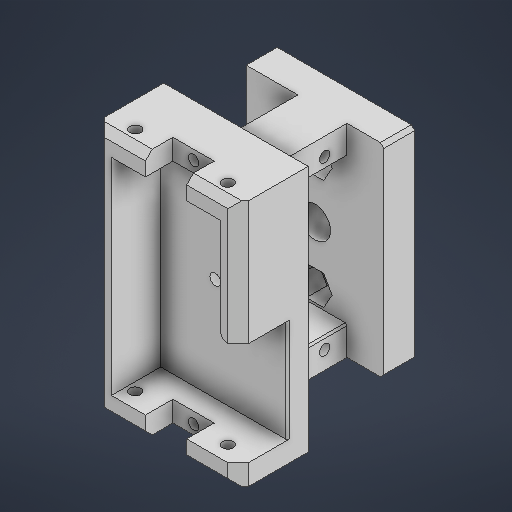
# Autodesk Inventor part: GA_Base
Saved by Autodesk Inventor 2025.2 (Build 292293000, 293)
## iProperties
Created: 2025-06-18
Part Number: GA_Base
Material: Generic
Document SubType Name: Modeling
Designer: Tiago
Density: 1 g/cm^3
Appearance: Default
Author: Tiago
Autodesk Inventor part; units mm, degrees
sketch "Sketch1" plane through (0, 0, 0) normal (0, 0, 1) x (1, 0, 0)
  line L0 (-15.9, 30) -> (15.9, 30)
  line L1 (15.9, 30) -> (15.9, -30)
  line L2 (15.9, -30) -> (-15.9, -30)
  line L3 (-15.9, -30) -> (-15.9, 30)
  line L4 (-21, -36) -> (21, -36)
  line L5 (21, -36) -> (21, 36)
  line L6 (21, 36) -> (-21, 36)
  line L7 (-21, 36) -> (-21, -36)
  circle A0 centre (0, 0) radius 1.575
  point P0 (15.9, 0)
  point P1 (0, 30)
  point P2 (0, 36)
  point P3 (-21, 0)
  dimension "d0" = 31.8
  dimension "d1" = 60
  dimension "d4" = 42
  dimension "d5" = 72
  dimension "d40" = 3.15
  constraints: 16 end point, 5 coincident, 4 midpoint, 4 parallel, 2 horizontal, 2 horizontal alignment, 2 perpendicular, 2 vertical alignment, 1 centre point
  measures "d0" distance of L1.end L2.end
  measures "d1" distance of L0.end L1.end
  measures "d4" distance of L5.end L6.end
  measures "d5" distance of L4.end L5.end
  measures "d40" diameter of A0
extrude "Extrusion1" add sketch "Sketch1" along normal blind 20.35 contours L7 L6 L5 L4
extrude "Extrusion2" add sketch "Sketch1" along normal blind 6 contours L0 L1 L2 L3
chamfer "Chamfer1" distance 3 angle 45 2 edges at (21, 0, 20.35) (-21, 0, 20.35)
chamfer "Chamfer2" distance 2 angle 45 2 edges at (0, -36, 20.35) (0, 36, 20.35)
sketch "Sketch2" plane through (0, 0, 20.35) normal (0, 0, 1) x (1, 0, 0)
  line L0 (-18, 34) -> (18, 34) projected
  line L1 (18, 34) -> (18, -34) projected
  line L2 (18, -34) -> (-18, -34) projected
  line L3 (-18, -34) -> (-18, 34) projected
  line L4 (15.9, 30) -> (-15.9, 30) projected
  line L5 (-15.9, 30) -> (-15.9, -30) projected
  line L6 (-15.9, -30) -> (15.9, -30) projected
  line L7 (15.9, -30) -> (15.9, 30) projected
  circle A0 centre (0, -33.25) radius 1.5
  line L8 (-6, -38) -> (6, -38)
  line L9 (6, -38) -> (6, -30)
  line L10 (6, -30) -> (-6, -30)
  line L11 (-6, -30) -> (-6, -38)
  line L12 (-3.2097, 0) -> (3.2097, 0) construction
  circle A1 centre (0, 33.25) radius 1.5
  line L13 (-6, 38) -> (6, 38)
  line L14 (6, 38) -> (6, 30)
  line L15 (6, 30) -> (-6, 30)
  line L16 (-6, 30) -> (-6, 38)
  point P0 (0, 0)
  point P1 (0, -30)
  point P2 (0, -30)
  point P3 (0, 0)
  point P4 (0, 30)
  point P5 (0, 30)
  dimension "d16" = 3
  dimension "d18" = 33.25
  dimension "d19" = 12
  dimension "d20" = 8
  constraints: 18 end point, 7 symmetric about line, 3 coincident, 3 midpoint, 2 centre point, 2 horizontal, 2 parallel, 2 vertical alignment, 1 perpendicular, 1 other
  measures "d16" diameter of A0
  measures "d18" distance of point (0, 0) A0.centre
  measures "d19" distance between parallel lines of L11 L9
  measures "d20" distance of L8.end L9.end
extrude "Extrusion3" cut sketch "Sketch2" against normal blind 8 contours L16 L13 L14 L0 A1 | L0 A1 L14 L4 L16 | L11 L6 L9 L2 A0 | L2 A0 L9 L8 L11
extrude "Extrusion4" cut sketch "Sketch2" against normal blind 18 contours A1 L0 | L0 A1 | A0 L2 | L2 A0
ref_plane "Work Plane1" through (15.75, -36, 0) normal (1, 0, 0) x (0, 0, -1)
sketch "Sketch4" plane through (15.75, -36, 0) normal (1, 0, 0) x (0, 0, -1)
  line L0 (-18.35, 72) -> (0, 72) projected
  line L1 (0, 72) -> (0, 0) projected
  line L2 (0, 0) -> (-18.35, 0) projected
  line L3 (-18.35, 0) -> (-20.35, 2) projected
  line L4 (-20.35, 2) -> (-20.35, 6) projected
  line L5 (-20.35, 66) -> (-20.35, 70) projected
  line L6 (-20.35, 70) -> (-18.35, 72) projected
  line L7 (-20.35, 6) -> (-6, 6)
  line L8 (-6, 6) -> (-6, 36)
  line L9 (-6, 6) -> (-6, 66) projected
  line L10 (-6, 36) -> (-20.35, 36)
  line L11 (-20.35, 36) -> (-20.35, 6)
  line L12 (-20.35, 6) -> (-6, 6) projected
  line L13 (-6, 6) -> (-6, 66) projected
  line L14 (-6, 66) -> (-20.35, 66) projected
  point P0 (0, 36)
  dimension "d26" = 30
  constraints: 8 end point, 1 collinear, 1 horizontal, 1 midpoint
  measures "d26" distance of L7.end L8.end
extrude "Extrusion5" cut sketch "Sketch4" along normal up to surface (5.25 mm away) contours L8 L7 L11 L10
fillet "Fillet1" radius 2 1 edges at (15.9, 0, 13.175)
chamfer "Chamfer3" distance 0.5 angle 45 1 edges at (21, -15, 6)
ref_plane "Work Plane2" through (-21, 33, 0) normal (0, 1, 0) x (1, 0, 0)
sketch "Sketch6" plane through (-21, 33, 0) normal (0, 1, 0) x (1, 0, 0)
  line L0 (15, -12.35) -> (15, -20.35) projected
  line L1 (15, -20.35) -> (3, -20.35) projected
  line L2 (3, -20.35) -> (0, -17.35) projected
  line L3 (0, -17.35) -> (0, 0) projected
  line L4 (0, 0) -> (42, 0) projected
  line L5 (42, 0) -> (42, -17.35) projected
  line L6 (42, -17.35) -> (39, -20.35) projected
  line L7 (39, -20.35) -> (27, -20.35) projected
  line L8 (27, -20.35) -> (27, -12.35) projected
  line L9 (27, -12.35) -> (22.479, -12.35) projected
  line L10 (22.479, -12.35) -> (22.479, -2.35) projected
  line L11 (22.479, -2.35) -> (19.521, -2.35) projected
  line L12 (19.521, -2.35) -> (19.521, -12.35) projected
  line L13 (19.521, -12.35) -> (15, -12.35) projected
  circle A0 centre (34.45, -15.85) radius 1.575
  circle A1 centre (7.55, -15.85) radius 1.575
  point P0 (21, 0)
  dimension "Veio" = 3.15
  dimension "d34" = 3.15
  dimension "d35" = 4.5
  dimension "d36" = 7.55
  dimension "d37" = 7.55
  constraints: 2 centre point, 1 horizontal alignment
  measures "Veio" diameter of A0
  measures "d34" diameter of A1
  measures "d35" distance from line of L7 A0.centre
  measures "d36" distance from line of L5 A0.centre
  measures "d37" distance from line of L3 A1.centre
extrude "Extrusion6" cut sketch "Sketch6" along normal through all both and the other way through all contours A0 | A1
sketch "Sketch7" plane through (0, 0, 0) normal (0, 0, -1) x (-1, 0, 0)
  line L0 (20, -20.5) -> (-20, -20.5)
  line L1 (-20, -20.5) -> (-20, 20.5)
  line L2 (-20, 20.5) -> (20, 20.5)
  line L3 (20, 20.5) -> (20, -20.5)
  line L4 (-9.3, -29.5) -> (20, -29.5)
  line L5 (20, -29.5) -> (20, 29.5)
  line L6 (20, 29.5) -> (-9.3, 29.5)
  line L7 (-9.3, 29.5) -> (-9.3, -29.5)
  line L8 (-9.3, -21) -> (20, -21)
  line L9 (-9.3, 21) -> (20, 21)
  line L10 (5, 29.5) -> (5, 21)
  line L11 (5, -21) -> (5, -29.5)
  point P0 (0, 0)
  point P1 (-20, 0)
  point P2 (0, -20.5)
  point P3 (20, 0)
  point P4 (20, 0)
  point P5 (-9.3, 20.5)
  point P6 (-9.3, -20.5)
  dimension "d41" = 41
  dimension "d42" = 40
  dimension "d43" = 9
  dimension "d44" = 9
  dimension "d47" = 10.7
  dimension "d101" = 0.5
  dimension "d102" = 0.5
  dimension "d122" = 15
  dimension "d123" = 15
  constraints: 24 end point, 8 point on line, 6 perpendicular, 4 midpoint, 4 parallel, 2 horizontal, 1 coincident, 1 horizontal alignment, 1 vertical alignment
  measures "d41" distance of L0.end L1.end
  measures "d42" distance of L1.end L2.end
  measures "d43" distance between parallel lines of L4 L0
  measures "d44" distance between parallel lines of L6 L2
  measures "d47" distance between parallel lines of L7 L1
  measures "d101" distance between parallel lines of L2 L9
  measures "d102" distance between parallel lines of L0 L8
  measures "d122" distance between parallel lines of L5 L11
  measures "d123" distance between parallel lines of L5 L10
extrude "Extrusion7" add sketch "Sketch7" along normal blind 23 contours L8 L11 L4 L7 | L7 L6 L10 L9
ref_plane "Work Plane3" through (0, 0, -23) normal (0, 0, -1) x (-1, 0, 0)
sketch "Sketch8" plane through (0, 0, -23) normal (0, 0, -1) x (-1, 0, 0)
  line L0 (20, -29.5) -> (-20, -29.5)
  line L1 (-20, -29.5) -> (-20, 29.5)
  line L2 (-20, 29.5) -> (20, 29.5)
  line L3 (20, 29.5) -> (20, -29.5)
  point P0 (0, 0)
  point P1 (-20, 0)
  point P2 (0, 29.5)
  dimension "d51" = 40
  dimension "d52" = 59
  constraints: 8 end point, 2 midpoint, 2 parallel, 1 horizontal, 1 horizontal alignment, 1 perpendicular, 1 vertical alignment
  measures "d51" distance of L1.end L2.end
  measures "d52" distance of L2.end L0.start
extrude "Extrusion8" add sketch "Sketch8" along normal blind 9
ref_plane "Work Plane4" through (9.3, -29.5, 0) normal (1, 0, 0) x (0, 0, -1)
sketch "Sketch9" plane through (9.3, -29.5, 0) normal (1, 0, 0) x (0, 0, -1)
  circle A0 centre (6.5, 5.2) radius 1.5
  circle A1 centre (6.5, 53.8) radius 1.5
  circle A2 centre (16.5, 53.8) radius 1.5
  circle A3 centre (16.5, 5.2) radius 1.5
  point P0 (0, 29.5)
  point P1 (11.2, 29.5)
  dimension "mss" = 3
  dimension "d57" = 3
  dimension "d58" = 3
  dimension "d59" = 3
  dimension "d60" = 24.3
  dimension "d61" = 24.3
  dimension "d62" = 24.3
  dimension "d63" = 24.3
  dimension "d64" = 10
  dimension "d65" = 10
  dimension "d66" = 11.2
  dimension "d67" = 4.7
  dimension "d68" = 4.7
  constraints: 4 centre point, 1 horizontal alignment
  measures "mss" diameter of A0
  measures "d57" diameter of A3
  measures "d58" diameter of A2
  measures "d59" diameter of A1
  measures "d60" vertical distance of A3.centre point (0, 29.5)
  measures "d61" vertical distance of point (0, 29.5) A0.centre
  measures "d62" vertical distance of point (0, 29.5) A1.centre
  measures "d63" vertical distance of point (0, 29.5) A2.centre
  measures "d64" distance of A0.centre A3.centre
  measures "d65" distance of A2.centre A1.centre
  measures "d66" distance of point (0, 29.5) point (11.2, 29.5)
  measures "d67" horizontal distance of A1.centre point (11.2, 29.5)
  measures "d68" horizontal distance of A0.centre point (11.2, 29.5)
extrude "Extrusion9" cut sketch "Sketch9" against normal through all
ref_plane "Work Plane5" through (-20, 29.5, 0) normal (0, 1, 0) x (1, 0, 0)
sketch "Sketch12" plane through (0, 0, -23) normal (0, 0, 1) x (1, 0, 0)
  circle A0 centre (0, 16) radius 2.5
  circle A1 centre (0, -16) radius 2.5
  circle A2 centre (0, 0) radius 4.5
  line L0 (-5, -16) -> (-2.5, -11.6699)
  line L1 (-2.5, -11.6699) -> (2.5, -11.6699)
  line L2 (2.5, -11.6699) -> (5, -16)
  line L3 (5, -16) -> (2.5, -20.3301)
  line L4 (2.5, -20.3301) -> (-2.5, -20.3301)
  line L5 (-2.5, -20.3301) -> (-5, -16)
  line L6 (-5, 16) -> (-2.5, 20.3301)
  line L7 (-2.5, 20.3301) -> (2.5, 20.3301)
  line L8 (2.5, 20.3301) -> (5, 16)
  line L9 (5, 16) -> (2.5, 11.6699)
  line L10 (2.5, 11.6699) -> (-2.5, 11.6699)
  line L11 (-2.5, 11.6699) -> (-5, 16)
  dimension "d103" = 32
  dimension "d104" = 5
  dimension "d105" = 5
  dimension "d106" = 9
  dimension "d107" = 16
  dimension "d108" = 10
  dimension "d109" = 10
  constraints: 24 end point, 3 centre point, 3 coincident, 2 horizontal alignment, 2 vertical alignment, 26 other
  measures "d103" distance of A1.centre A0.centre
  measures "d104" diameter of A0
  measures "d105" diameter of A1
  measures "d106" diameter of A2
  measures "d107" distance of point (0, 0) A0.centre
  measures "d108" distance of L6.start L8.end
  measures "d109" distance of L2.end L0.start
extrude "Extrusion13" cut sketch "Sketch12" against normal up to surface (9 mm away) contours A0 | A1 | A2
extrude "Extrusion14" cut sketch "Sketch12" against normal blind 6 contours L0 L1 L2 L3 L4 L5 | L6 L7 L8 L9 L10 L11
chamfer "Chamfer4" distance 0.5 angle 45 2 edges at (9.3, 21, -11.5) (9.3, -21, -11.5)
chamfer "Chamfer5" distance 1 angle 45 2 edges at (20, 29.5, -27.5) (20, -29.5, -27.5)
extrude "Extrusion15" add sketch "Sketch1" along normal blind 1.5 contours A0
equation "\"d40\" = Veio"
equation "\"d34\" = Veio"
equation "\"d57\" = mss"
equation "\"d58\" = mss"
equation "\"d59\" = mss"
body "Solid1"
